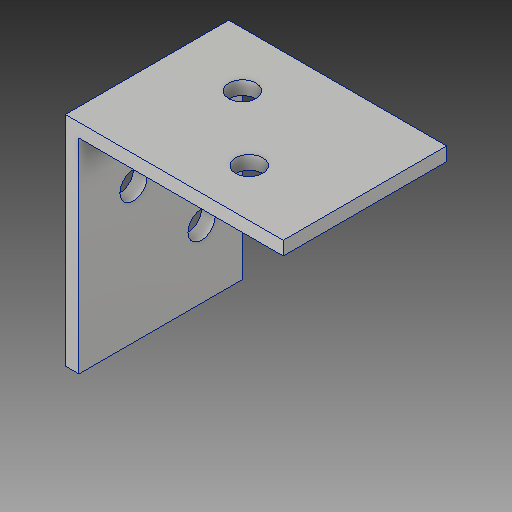
# Autodesk Inventor part: 15102898-16-P-0802
Saved by Autodesk Inventor 2017 (Build 210142000, 142)
## iProperties
Created: 2016-10-10
Part Number: 15102898-16-P-0802
Material: Aluminum 6061
Document SubType Name: Modeling
Designer: gus
Density: 2.7 g/cm^3
Appearance: Aluminum - Flat
Mass: 31.0609 g
Surface Area: 83.6692 cm^2
Volume: 11.504 cm^3
Author: gus
Autodesk Inventor part; units mm, degrees
ref_plane "YZ Plane" through (0, 0, 0) normal (1, 0, 0) x (0, 1, 0)
ref_plane "XZ Plane" through (0, 0, 0) normal (0, 1, 0) x (-1, 0, 0)
ref_plane "XY Plane" through (0, 0, 0) normal (0, 0, 1) x (1, 0, 0)
sketch "Sketch1" plane through (0, 0, 0) normal (0, 0, 1) x (1, 0, 0)
  line L0 (0, 0) -> (50.8, 0)
  line L1 (50.8, 0) -> (50.8, -3.175)
  line L2 (50.8, -3.175) -> (3.175, -3.175)
  line L3 (3.175, -3.175) -> (3.175, -50.8)
  line L4 (3.175, -50.8) -> (0, -50.8)
  line L5 (0, -50.8) -> (0, 0)
  dimension "d0" = 3.175
  dimension "d1" = 3.175
  dimension "d2" = 50.8
  dimension "d3" = 50.8
  constraints: 12 end point, 5 perpendicular, 1 horizontal
  measures "d0" distance of L3.end L4.end
  measures "d1" distance of L0.end L1.end
  measures "d2" distance of L0.start L0.end
  measures "d3" distance of L4.end L0.start
extrude "Extrusion1" add sketch "Sketch1" along normal blind 38.1
sketch "Sketch2" plane through (0, -50.8, 0) normal (-1, 0, 0) x (0, 0, 1)
  circle A0 centre (25.4, 31.75) radius 3.175
  circle A1 centre (9.525, 15.875) radius 3.175
  line L0 (0, 0) -> (0, 50.8) projected
  line L1 (0, 50.8) -> (38.1, 50.8) projected
  line L2 (0, 0) -> (38.1, 0) projected
  dimension "d6" = 6.35
  dimension "d7" = 6.35
  dimension "d8" = 9.525
  dimension "d9" = 25.4
  dimension "d12" = 19.05
  dimension "d13" = 15.875
  constraints: 2 centre point
  measures "d6" diameter of A1
  measures "d7" diameter of A0
  measures "d8" distance from line of L0 A1.centre
  measures "d9" distance from line of L0 A0.centre
  measures "d12" distance from line of L1 A0.centre
  measures "d13" distance from line of L2 A1.centre
extrude "Extrusion2" cut sketch "Sketch2" against normal blind 3.175
sketch "Sketch3" plane through (0, 0, 0) normal (0, 1, 0) x (1, 0, 0)
  circle A0 centre (15.875, -12.7) radius 3.175
  circle A1 centre (31.75, -26.9875) radius 3.175
  line L0 (0, 0) -> (50.8, 0) projected
  line L1 (50.8, -38.1) -> (0, -38.1) projected
  line L2 (50.8, 0) -> (50.8, -38.1) projected
  line L3 (0, 0) -> (0, -38.1) projected
  dimension "d14" = 6.35
  dimension "d15" = 6.35
  dimension "d16" = 12.7
  dimension "d17" = 11.1125
  dimension "d18" = 19.05
  dimension "d19" = 15.875
  constraints: 2 centre point
  measures "d14" diameter of A0
  measures "d15" diameter of A1
  measures "d16" distance from line of L0 A0.centre
  measures "d17" distance from line of L1 A1.centre
  measures "d18" distance from line of A1.centre L2
  measures "d19" distance from line of L3 A0.centre
extrude "Extrusion3" cut sketch "Sketch3" against normal blind 3.175 contours A0 | A1
body "Solid1"
